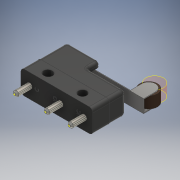
# Autodesk Inventor part: 49-0006
Saved by Autodesk Inventor 2018 (Build 220112000, 112)
## iProperties
Created: 2020-02-12
Part Number: 49-0006
Material: Generic
Document SubType Name: Modeling
Designer: Bradley
Density: 1 g/cm^3
Appearance: Smooth - Black
Author: Bradley
Autodesk Inventor part; units mm, degrees
ref_plane "YZ Plane" through (0, 0, 0) normal (1, 0, 0) x (0, 1, 0)
ref_plane "XZ Plane" through (0, 0, 0) normal (0, 1, 0) x (-1, 0, 0)
ref_plane "XY Plane" through (0, 0, 0) normal (0, 0, 1) x (1, 0, 0)
sketch "Sketch1" plane through (0, 0, 0) normal (0, 0, 1) x (1, 0, 0)
  line L0 (9.9, -2.3) -> (-9.9, -2.3)
  line L1 (-9.9, -2.3) -> (-9.9, 2.3)
  line L2 (-9.9, 2.3) -> (9.9, 2.3)
  line L3 (9.9, 2.3) -> (9.9, -2.3)
  line L4 (9.9, -2.3) -> (-9.9, 2.3) construction
  line L5 (-9.9, -2.3) -> (9.9, 2.3) construction
  circle A0 centre (4.75, 0) radius 1.15
  line L6 (-6, 0) -> (-3.5, 0) construction
  line L7 (-4.85, -1.15) -> (-4.65, -1.15)
  line L8 (-4.65, 1.15) -> (-4.85, 1.15)
  arc A1 (-4.85, 1.15) -> (-4.85, -1.15) centre (-4.85, 0) ccw
  arc A2 (-4.65, -1.15) -> (-4.65, 1.15) centre (-4.65, 0) ccw
  line L9 (4.75, 0) -> (-4.75, 0) construction
  line L10 (9.85, 2.3) -> (9.85, 6.9)
  line L11 (9.85, 6.9) -> (-9.85, 6.9)
  line L12 (-9.85, 6.9) -> (-9.85, 2.3)
  line L13 (-7.25, 8.7) -> (13.05, 8.7)
  line L14 (13.05, 8.7) -> (13.05, 8.5)
  line L15 (13.05, 8.5) -> (-7.25, 8.5)
  line L16 (-7.25, 8.5) -> (-7.25, 8.7)
  circle A3 centre (11.15, 11.8) radius 2.4
  line L17 (11.15, 11.8) -> (-7.25, 8.5) construction
  line L18 (-7.25, 8.5) -> (10.6284, 13.96) construction
  circle A4 centre (10.6284, 13.96) radius 2.4
  circle A5 centre (11.15, 11.8) radius 1.9 construction
  point P0 (0, 0)
  point P1 (0, 0)
  point P2 (0, 6.9)
  point P3 (0, 0)
  dimension "d0" = 19.8
  dimension "d1" = 4.6
  dimension "d2" = 2.3
  dimension "d3" = 2.5
  dimension "d4" = 9.5
  dimension "d7" = 19.7
  dimension "d8" = 6.9
  dimension "d11" = 6.4
  dimension "d12" = 11.8
  dimension "d13" = 4.8
  dimension "d14" = 8.7
  dimension "d15" = 0.2
  dimension "d16" = 12
  dimension "d21" = 2.16
  dimension "d24" = 3.8
  constraints: 40 end point, 7 midpoint, 6 centre point, 6 point on circle, 5 parallel, 5 tangent, 4 perpendicular, 4 point on line, 3 horizontal, 2 coincident, 2 equal radius, 1 collinear, 1 equal length, 1 vertical, 1 vertical alignment
  measures "d0" distance of L1.end L2.end
  measures "d1" distance of L0.end L1.end
  measures "d2" diameter of A0
  measures "d3" distance of L6.start L6.end
  measures "d4" distance of L9.start L9.end
  measures "d7" distance of L10.end L11.end
  measures "d8" distance from line of L9.start L11
  measures "d11" horizontal distance of L9.start L17.start
  measures "d12" vertical distance of L9.start L17.start
  measures "d13" diameter of A3
  measures "d14" distance from line of L9.start L13
  measures "d15" distance of L13.end L14.end
  measures "d16" distance from line of L9.start L16
  measures "d21" vertical distance of L17.start L18.end
  measures "d24" diameter of A5
extrude "Extrusion1" add sketch "Sketch1" along normal mid plane 6.4 contours L0 L1 L2 L3
extrude "Extrusion2" add sketch "Sketch1" along normal mid plane 6.3 contours L2 L12 L11 L10
extrude "Extrusion3" add sketch "Sketch1" along normal mid plane 3.6 contours L13 L14 L15 L16
extrude "Extrusion4" add sketch "Sketch1" along normal mid plane 3.2 contours A3 A4 | A4 A3 picked at (11.2706, 10.9018) picked at (10.8948, 12.4454)
surface extrude "ExtrusionSrf1" sketch "Sketch1" along normal mid plane 3.2 shown yes curves A4
sketch "Sketch2" plane through (0, 0, 1.8) normal (0, 0, 1) x (1, 0, 0)
  circle A0 centre (11.15, 11.8) radius 2.4 projected
  line L0 (13.05, 8.7) -> (-7.25, 8.7) projected
  line L1 (-7.25, 8.7) -> (-7.25, 8.5) projected
  line L2 (-7.25, 8.5) -> (13.05, 8.5) projected
  line L3 (13.05, 8.5) -> (13.05, 8.7) projected
  line L4 (13.05, 8.7) -> (13.05, 11.8)
  arc A1 (13.05, 11.8) -> (9.25, 11.8) centre (11.15, 11.8) ccw
  line L5 (9.25, 11.8) -> (9.25, 8.7)
  line L6 (9.85, 2.3) -> (9.85, 6.9) projected
  line L7 (9.85, 6.9) -> (-9.85, 6.9) projected
  line L8 (-9.85, 6.9) -> (-9.85, 2.3) projected
  line L9 (9.85, 2.3) -> (-9.85, 2.3) projected
  line L10 (-9.85, 6.9) -> (9.85, 6.9) projected
  line L11 (-9.85, 6.9) -> (-9.85, 10.2)
  line L12 (-9.85, 10.2) -> (-0.55, 10.2)
  line L13 (-0.55, 10.2) -> (-0.55, 6.9)
  point P0 (0, 0)
  dimension "d27" = 10.2
  dimension "d54" = 9.3
  constraints: 10 end point, 3 perpendicular, 2 point on circle, 2 point on line, 2 tangent, 2 vertical, 1 centre point, 1 concentric
  measures "d27" distance from line of point (0, 0) L12
  measures "d54" distance of L11.end L12.end
extrude "Extrusion5" add sketch "Sketch2" against normal up to surface (0.2 mm away) contours L5 A1 L4 A0 | A0 L4 L0 L5 picked at (11.15, 11)
extrude "Extrusion6" add sketch "Sketch2" along normal up to surface (1.35 mm away) contours L13 L2 L1 L0 | L0 L1 L2 L13 L7 L11 L12
mirror "Mirror1" about plane through (0, 0, 0) normal (0, 0, 1) of "Extrusion6"
fillet "Fillet1" radius 1 13 edges at (-9.9, 0, 3.2) (-9.85, 6.25, 3.15) (4.65, 6.9, 3.15) (9.85, 6.9, 0) (9.85, 4.6, 3.15) (9.9, 0, 3.2) (9.85, 4.6, -3.15) (9.9, 0, -3.2) (-0.55, 10.2, 2.475) (-0.55, 10.2, -2.475) (-9.85, 6.25, -3.15) (4.65, 6.9, -3.15) (-9.9, 0, -3.2)
fillet "Fillet1" radius 0.8 6 edges at (-5.2, 10.2, -3.15) (-0.55, 8.55, -3.15) (-0.55, 8.55, 3.15) (-5.2, 10.2, 3.15) (-9.85, 10.2, -2.475) (-9.85, 10.2, 2.475)
fillet "Fillet1" radius 0.4 2 edges at (-0.55, 6.9, 2.475) (-0.55, 6.9, -2.475)
mirror "Mirror2" about plane through (0, 0, 0) normal (0, 0, 1) of "Extrusion5"
sketch "Sketch3" plane through (-8.9, -2.3, -3.2) normal (0, -1, 0) x (1, 0, 0)
  circle A0 centre (1.4, 3.2) radius 0.735
  circle A1 centre (9.9, 3.2) radius 0.735
  circle A2 centre (16.4, 3.2) radius 0.735
  line L0 (1.4, 3.2) -> (16.4, 3.2) construction
  point P0 (8.9, 3.2)
  point P1 (8.9, 3.2)
  dimension "d34" = 1.47
  dimension "d35" = 15
  dimension "d36" = 1
  constraints: 3 centre point, 2 end point, 2 equal radius, 1 coincident, 1 horizontal, 1 midpoint, 1 point on line
  measures "d34" diameter of A0
  measures "d35" distance of L0.start L0.end
  measures "d36" distance of point (8.9, 3.2) A1.centre
extrude "Extrusion7" add sketch "Sketch3" along normal blind 4.1
chamfer "Chamfer1" distance 0.4 angle 45 3 edges at (-8.235, -6.4, 0) (0.265, -6.4, 0) (6.765, -6.4, 0)
sketch "Sketch4" plane through (-8.9, -2.3, -3.2) normal (0, -1, 0) x (1, 0, 0)
  circle A0 centre (9.9, 3.2) radius 0.735 projected
  circle A1 centre (1.4, 3.2) radius 0.735 projected
  circle A2 centre (16.4, 3.2) radius 0.735 projected
  arc A3 (-1, 1) -> (0, 0) centre (0, 1) ccw projected
  line L0 (17.8, 0) -> (0, 0) projected
  arc A4 (17.8, 0) -> (18.8, 1) centre (17.8, 1) ccw projected
  line L1 (18.8, 1) -> (18.8, 5.4) projected
  arc A5 (18.8, 5.4) -> (17.8, 6.4) centre (17.8, 5.4) ccw projected
  line L2 (0, 6.4) -> (17.8, 6.4) projected
  arc A6 (0, 6.4) -> (-1, 5.4) centre (0, 5.4) ccw projected
  line L3 (-1, 5.4) -> (-1, 1) projected
  line L4 (17.8, 0) -> (0, 0) construction
  line L5 (3.9, 0) -> (3.9, 6.4) construction
  line L6 (8.9, 0) -> (8.9, 6.4) construction
  line L7 (0, 6.4) -> (17.8, 6.4) construction
  line L8 (15.4, 0) -> (15.4, 6.4) construction
  spline S0 degree 2 poles (3.9178, 3.279) (3.9178, 3.1818) (3.8522, 3.0173) (3.7865, 2.9573) knots 0 0 0 1 2 2 2
  spline S1 degree 2 poles (3.7865, 2.9573) (3.7217, 2.8973) (3.5272, 2.8317) (3.4008, 2.8317) knots 0 0 0 1 2 2 2
  spline S2 degree 2 poles (3.4008, 2.8317) (3.2752, 2.8317) (3.0888, 2.8957) (3.0199, 2.9565) knots 0 0 0 1 2 2 2
  spline S3 degree 2 poles (3.0199, 2.9565) (2.9527, 3.0165) (2.8822, 3.1801) (2.8822, 3.2814) knots 0 0 0 1 2 2 2
  spline S4 degree 2 poles (2.8822, 3.2814) (2.8822, 3.3317) (2.8968, 3.42) (2.9081, 3.4573) knots 0 0 0 1 2 2 2
  spline S5 degree 2 poles (2.9081, 3.4573) (2.9186, 3.4897) (2.9486, 3.557) (2.9665, 3.5902) knots 0 0 0 1 2 2 2
  line L9 (2.9665, 3.5902) -> (3.1269, 3.5902)
  line L10 (3.1269, 3.5902) -> (3.1269, 3.5797)
  spline S6 degree 2 poles (3.1269, 3.5797) (3.1107, 3.5618) (3.0653, 3.5067) (3.0434, 3.467) knots 0 0 0 1 2 2 2
  spline S7 degree 2 poles (3.0434, 3.467) (3.0224, 3.4289) (2.9956, 3.339) (2.9956, 3.2806) knots 0 0 0 1 2 2 2
  spline S8 degree 2 poles (2.9956, 3.2806) (2.9956, 3.2166) (3.0483, 3.1024) (3.0985, 3.0594) knots 0 0 0 1 2 2 2
  spline S9 degree 2 poles (3.0985, 3.0594) (3.1496, 3.0173) (3.3044, 2.9703) (3.4008, 2.9703) knots 0 0 0 1 2 2 2
  spline S10 degree 2 poles (3.4008, 2.9703) (3.5037, 2.9703) (3.652, 3.0197) (3.7031, 3.0626) knots 0 0 0 1 2 2 2
  spline S11 degree 2 poles (3.7031, 3.0626) (3.7525, 3.1048) (3.8028, 3.2174) (3.8028, 3.2806) knots 0 0 0 1 2 2 2
  spline S12 degree 2 poles (3.8028, 3.2806) (3.8028, 3.3382) (3.7744, 3.4362) (3.7533, 3.4743) knots 0 0 0 1 2 2 2
  spline S13 degree 2 poles (3.7533, 3.4743) (3.7323, 3.5108) (3.6885, 3.5651) (3.6731, 3.5805) knots 0 0 0 1 2 2 2
  line L11 (3.6731, 3.5805) -> (3.6731, 3.5902)
  line L12 (3.6731, 3.5902) -> (3.8319, 3.5902)
  spline S14 degree 2 poles (3.8319, 3.5902) (3.8473, 3.557) (3.8757, 3.4986) (3.8887, 3.4573) knots 0 0 0 1 2 2 2
  spline S15 degree 2 poles (3.8887, 3.4573) (3.9032, 3.4135) (3.9178, 3.339) (3.9178, 3.279) knots 0 0 0 1 2 2 2
  line L13 (8.9, 3.0712) -> (8.9, 2.922)
  line L14 (8.9, 2.922) -> (8.0378, 2.4796)
  line L15 (8.0378, 2.4796) -> (8.9, 2.4796)
  line L16 (8.9, 2.4796) -> (8.9, 2.3556)
  line L17 (8.9, 2.3556) -> (7.9, 2.3556)
  line L18 (7.9, 2.3556) -> (7.9, 2.5444)
  line L19 (7.9, 2.5444) -> (8.6917, 2.9472)
  line L20 (8.6917, 2.9472) -> (7.9, 2.9472)
  line L21 (7.9, 2.9472) -> (7.9, 3.0712)
  line L22 (7.9, 3.0712) -> (8.9, 3.0712)
  spline S16 degree 2 poles (8.0143, 3.9812) (8.0807, 4.0379) (8.2752, 4.1011) (8.4, 4.1011) knots 0 0 0 1 2 2 2
  spline S17 degree 2 poles (8.4, 4.1011) (8.5216, 4.1011) (8.7185, 4.0395) (8.7849, 3.9812) knots 0 0 0 1 2 2 2
  spline S18 degree 2 poles (8.7849, 3.9812) (8.8546, 3.9196) (8.9211, 3.7567) (8.9211, 3.6587) knots 0 0 0 1 2 2 2
  spline S19 degree 2 poles (8.9211, 3.6587) (8.9211, 3.5574) (8.8522, 3.3953) (8.7849, 3.3361) knots 0 0 0 1 2 2 2
  spline S20 degree 2 poles (8.7849, 3.3361) (8.7185, 3.2786) (8.5232, 3.217) (8.4, 3.217) knots 0 0 0 1 2 2 2
  spline S21 degree 2 poles (8.4, 3.217) (8.2744, 3.217) (8.0831, 3.2794) (8.0143, 3.337) knots 0 0 0 1 2 2 2
  spline S22 degree 2 poles (8.0143, 3.337) (7.9478, 3.3953) (7.8789, 3.5582) (7.8789, 3.6587) knots 0 0 0 1 2 2 2
  spline S23 degree 2 poles (7.8789, 3.6587) (7.8789, 3.7608) (7.9502, 3.9245) (8.0143, 3.9812) knots 0 0 0 1 2 2 2
  spline S24 degree 2 poles (8.4, 3.9626) (8.3011, 3.9626) (8.148, 3.9196) (8.0977, 3.8807) knots 0 0 0 1 2 2 2
  spline S25 degree 2 poles (8.0977, 3.8807) (8.0459, 3.841) (7.994, 3.7292) (7.994, 3.6595) knots 0 0 0 1 2 2 2
  spline S26 degree 2 poles (7.994, 3.6595) (7.994, 3.5874) (8.0442, 3.4788) (8.0977, 3.4374) knots 0 0 0 1 2 2 2
  spline S27 degree 2 poles (8.0977, 3.4374) (8.1488, 3.3977) (8.3028, 3.3556) (8.4, 3.3556) knots 0 0 0 1 2 2 2
  spline S28 degree 2 poles (8.4, 3.3556) (8.5969, 3.3556) (8.806, 3.5209) (8.806, 3.6595) knots 0 0 0 1 2 2 2
  spline S29 degree 2 poles (8.806, 3.6595) (8.806, 3.7981) (8.5969, 3.9626) (8.4, 3.9626) knots 0 0 0 1 2 2 2
  line L23 (15.4, 3.1449) -> (15.4, 2.9958)
  line L24 (15.4, 2.9958) -> (14.5378, 2.5533)
  line L25 (14.5378, 2.5533) -> (15.4, 2.5533)
  line L26 (15.4, 2.5533) -> (15.4, 2.4293)
  line L27 (15.4, 2.4293) -> (14.4, 2.4293)
  line L28 (14.4, 2.4293) -> (14.4, 2.6182)
  line L29 (14.4, 2.6182) -> (15.1917, 3.0209)
  line L30 (15.1917, 3.0209) -> (14.4, 3.0209)
  line L31 (14.4, 3.0209) -> (14.4, 3.1449)
  line L32 (14.4, 3.1449) -> (15.4, 3.1449)
  spline S30 degree 2 poles (15.4178, 3.7381) (15.4178, 3.6408) (15.3522, 3.4763) (15.2865, 3.4164) knots 0 0 0 1 2 2 2
  spline S31 degree 2 poles (15.2865, 3.4164) (15.2217, 3.3564) (15.0272, 3.2908) (14.9008, 3.2908) knots 0 0 0 1 2 2 2
  spline S32 degree 2 poles (14.9008, 3.2908) (14.7752, 3.2908) (14.5888, 3.3548) (14.5199, 3.4156) knots 0 0 0 1 2 2 2
  spline S33 degree 2 poles (14.5199, 3.4156) (14.4527, 3.4755) (14.3822, 3.6392) (14.3822, 3.7405) knots 0 0 0 1 2 2 2
  spline S34 degree 2 poles (14.3822, 3.7405) (14.3822, 3.7908) (14.3968, 3.8791) (14.4081, 3.9164) knots 0 0 0 1 2 2 2
  spline S35 degree 2 poles (14.4081, 3.9164) (14.4186, 3.9488) (14.4486, 4.016) (14.4665, 4.0493) knots 0 0 0 1 2 2 2
  line L33 (14.4665, 4.0493) -> (14.6269, 4.0493)
  line L34 (14.6269, 4.0493) -> (14.6269, 4.0387)
  spline S36 degree 2 poles (14.6269, 4.0387) (14.6107, 4.0209) (14.5653, 3.9658) (14.5434, 3.9261) knots 0 0 0 1 2 2 2
  spline S37 degree 2 poles (14.5434, 3.9261) (14.5224, 3.888) (14.4956, 3.7981) (14.4956, 3.7397) knots 0 0 0 1 2 2 2
  spline S38 degree 2 poles (14.4956, 3.7397) (14.4956, 3.6757) (14.5483, 3.5614) (14.5985, 3.5185) knots 0 0 0 1 2 2 2
  spline S39 degree 2 poles (14.5985, 3.5185) (14.6496, 3.4763) (14.8044, 3.4293) (14.9008, 3.4293) knots 0 0 0 1 2 2 2
  spline S40 degree 2 poles (14.9008, 3.4293) (15.0037, 3.4293) (15.152, 3.4788) (15.2031, 3.5217) knots 0 0 0 1 2 2 2
  spline S41 degree 2 poles (15.2031, 3.5217) (15.2525, 3.5639) (15.3028, 3.6765) (15.3028, 3.7397) knots 0 0 0 1 2 2 2
  spline S42 degree 2 poles (15.3028, 3.7397) (15.3028, 3.7972) (15.2744, 3.8953) (15.2533, 3.9334) knots 0 0 0 1 2 2 2
  spline S43 degree 2 poles (15.2533, 3.9334) (15.2323, 3.9699) (15.1885, 4.0241) (15.1731, 4.0395) knots 0 0 0 1 2 2 2
  line L35 (15.1731, 4.0395) -> (15.1731, 4.0493)
  line L36 (15.1731, 4.0493) -> (15.3319, 4.0493)
  spline S44 degree 2 poles (15.3319, 4.0493) (15.3473, 4.016) (15.3757, 3.9577) (15.3887, 3.9164) knots 0 0 0 1 2 2 2
  spline S45 degree 2 poles (15.3887, 3.9164) (15.4032, 3.8726) (15.4178, 3.7981) (15.4178, 3.7381) knots 0 0 0 1 2 2 2
  point P0 (8.9, 3.2)
  dimension "d55" = 5
  dimension "d56" = 6.5
  constraints: 6 end point, 4 point on line, 4 vertical, 3 midpoint, 1 parallel, 1 perpendicular
  measures "d55" distance between parallel lines of L6 L5
  measures "d56" distance between parallel lines of L8 L6
emboss "Emboss1" sketch "Sketch4" operation add depth 0.05 direction (0, 1, 0) contours S0 S1 S2 S3 S4 S5 L9 L10 S6 S7 S8 S9 S10 S11 S12 S13 L11 L12 S14 S15 | L13 L14 L15 L16 L17 L18 L19 L20 L21 L22 | S16 S17 S18 S19 S20 S21 S22 S23 | L23 L24 L25 L26 L27 L28 L29 L30 L31 L32 | S30 S31 S32 S33 S34 S35 L33 L34 S36 S37 S38 S39 S40 S41 S42 S43 L35 L36 S44 S45
body "Solid1"
body "Srf1"
